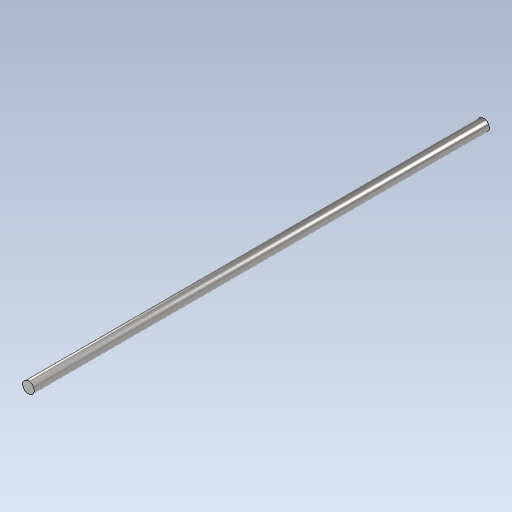
# Autodesk Inventor part: rod
Saved by Autodesk Inventor 2020 (Build 240168000, 168)
## iProperties
Created: 2020-05-14
Part Number: rod
Material: Ogólny
Document SubType Name: Modeling
Designer: blep
Density: 1 g/cm^3
Appearance: Domyślna
Author: blep
Autodesk Inventor part; units mm, degrees
ref_plane "YZ Plane" through (0, 0, 0) normal (1, 0, 0) x (0, 1, 0)
ref_plane "XZ Plane" through (0, 0, 0) normal (0, 1, 0) x (-1, 0, 0)
ref_plane "XY Plane" through (0, 0, 0) normal (0, 0, 1) x (1, 0, 0)
sketch "Szkic1" plane through (0, 0, 0) normal (0, 0, 1) x (1, 0, 0)
  circle A0 centre (-18.7, -17) radius 1.25 projected
  point P0 (0, 0)
  dimension "d0" = 100
extrude "Wyciągnięcie proste1" add sketch "Szkic1" along normal blind 100
